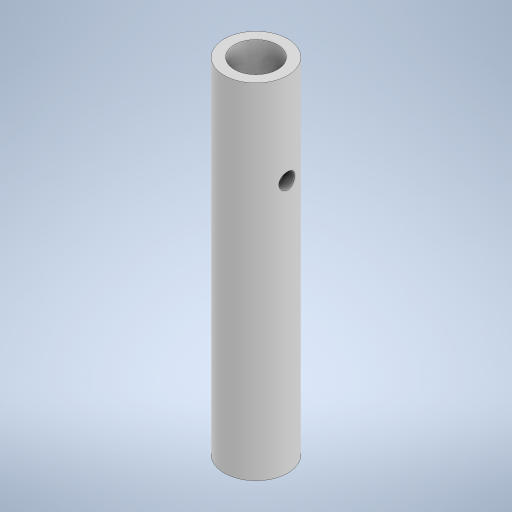
# Autodesk Inventor part: Valve Tube
Saved by Autodesk Inventor 2023 (Build 270158000, 158)
## iProperties
Created: 2023-02-13
Part Number: Valve Tube
Material: Generic
Document SubType Name: Modeling
Designer: tommy
Density: 1 g/cm^3
Appearance: Default
Author: tommy
Autodesk Inventor part; units mm, degrees
ref_plane "YZ Plane" through (0, 0, 0) normal (1, 0, 0) x (0, 1, 0)
ref_plane "XZ Plane" through (0, 0, 0) normal (0, 1, 0) x (-1, 0, 0)
ref_plane "XY Plane" through (0, 0, 0) normal (0, 0, 1) x (1, 0, 0)
sketch "Sketch1" plane through (0, 0, 0) normal (0, 1, 0) x (-1, 0, 0)
  circle A0 centre (0, 0) radius 1.0795
  circle A1 centre (0, 0) radius 1.5875
  dimension "d0" = 2.159
  dimension "d1" = 3.175
  constraints: 2 centre point, 2 coincident
  measures "d0" diameter of A0
  measures "d1" diameter of A1
extrude "Extrusion1" add sketch "Sketch1" along normal blind 17.272
sketch "Sketch2" plane through (0, 0, 0) normal (1, 0, 0) x (0, 1, 0)
  circle A0 centre (7.62, 0) radius 0.8382
  line L0 (17.272, -1.5875) -> (17.272, 1.5875) projected
  circle A1 centre (12.7, 0) radius 0.3969
  line L1 (17.272, 1.0795) -> (17.272, -1.0795) projected
  point P0 (0, 0)
  dimension "d4" = 1.6764
  dimension "d5" = 9.652
  dimension "d8" = 0.7937
  dimension "d9" = 4.572
  constraints: 2 centre point
  measures "d4" diameter of A0
  measures "d5" distance from line of L0 A0.centre
  measures "d8" diameter of A1
  measures "d9" distance from line of L1 A1.centre
extrude "Extrusion2" cut sketch "Sketch2" against normal blind 17.272 contours A0
extrude "Extrusion3" cut sketch "Sketch2" along normal blind 25.4 contours A1
body "Solid1"
